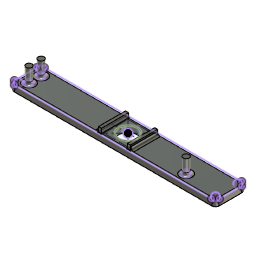
Front_Cover_OV3660 (Autodesk Fusion 360 design; units mm, degrees)
Autodesk Fusion 360 part; units mm, degrees
imported_body "Base Feature1" makes body 1
sketch "sketch 169" plane through (0, 0, 2) normal (0, 0, 1) x (-1, 0, 0)
  line L0 (-67.2527, -0.8) -> (-67.2527, -8.2)
  arc A0 (-67.2527, -8.2) -> (-66, -9.4527) centre (-66, -8.2) ccw
  line L1 (-66, -9.4527) -> (-0.8, -9.4527)
  arc A1 (-0.8, -9.4527) -> (0.4527, -8.2) centre (-0.8, -8.2) ccw
  line L2 (0.4527, -8.2) -> (0.4527, -0.8)
  arc A2 (0.4527, -0.8) -> (-0.8, 0.4527) centre (-0.8, -0.8) ccw
  line L3 (-0.8, 0.4527) -> (-66, 0.4527)
  arc A3 (-66, 0.4527) -> (-67.2527, -0.8) centre (-66, -0.8) ccw
  line L4 (-12, -7.75) -> (-15, -7.75)
  line L5 (-37.8, 0) -> (-37.8, -9)
  line L6 (-37.8, -9) -> (-39.8, -9)
  line L7 (-67.2527, -0.8) -> (-67.2527, -8.2)
  arc A4 (-67.2527, -8.2) -> (-66, -9.4527) centre (-66, -8.2) ccw
  line L8 (-66, -9.4527) -> (-0.8, -9.4527)
  arc A5 (-0.8, -9.4527) -> (0.4527, -8.2) centre (-0.8, -8.2) ccw
  line L9 (0.4527, -8.2) -> (0.4527, -0.8)
  arc A6 (0.4527, -0.8) -> (-0.8, 0.4527) centre (-0.8, -0.8) ccw
  line L10 (-0.8, 0.4527) -> (-66, 0.4527)
  arc A7 (-66, 0.4527) -> (-67.2527, -0.8) centre (-66, -0.8) ccw
  line L11 (-0.8, 0.4527) -> (-66, 0.4527)
  line L12 (-67.2527, -0.8) -> (-67.2527, -8.2)
  line L13 (-66, -9.4527) -> (-0.8, -9.4527)
  line L14 (0.4527, -8.2) -> (0.4527, -0.8)
  arc A8 (-0.8, -9.4527) -> (0.4527, -8.2) centre (-0.8, -8.2) ccw
  arc A9 (0.4527, -0.8) -> (-0.8, 0.4527) centre (-0.8, -0.8) ccw
  arc A10 (-66, 0.4527) -> (-67.2527, -0.8) centre (-66, -0.8) ccw
  arc A11 (-67.2527, -8.2) -> (-66, -9.4527) centre (-66, -8.2) ccw
  line L15 (0.1, -0.5) -> (-60.4, -0.5) construction
  line L16 (-60.4, -0.5) -> (-60.4, -8.5) construction
  line L17 (-60.4, -8.5) -> (0.1, -8.5) construction
  line L18 (0.1, -8.5) -> (0.1, -0.5) construction
  circle A12 centre (-33.4, -4.5) radius 3.1
  line L19 (0.1, -4.5) -> (-60.4, -4.5) construction
  line L20 (-0.8, -8.2) -> (-66, -0.8) construction
  line L21 (-66, -8.2) -> (-0.8, -0.8) construction
  constraint coincident A2.end L3.start
  constraint coincident L3.end A3.start
  constraint coincident L0.start A3.end
  constraint coincident L0.end A0.start
  constraint coincident A0.end L1.start
  constraint coincident L1.end A1.start
  constraint coincident A1.end L2.start
  constraint coincident L2.end A2.start
  constraint tangent L8 A8
  constraint tangent L14 A9
  constraint tangent L11 A9
  constraint tangent L11 A10
  constraint tangent L12 A11
  constraint horizontal L15
  constraint vertical L16
  constraint horizontal L17
  constraint vertical L18
  constraint coincident L15.start L18.end
  constraint midpoint L18 L19.start
  constraint midpoint L16 L19.end
  constraint coincident A12.centre L19
  constraint coincident A1.centre A5.centre
  constraint coincident A3.centre A7.centre
  constraint coincident A0.centre A4.centre
  constraint coincident A2.centre A6.centre
  constraint coincident A12.centre L21
  constraint coincident A12.centre L20
extrude "Extrude1" add sketch "sketch 169" against normal blind 2 separate body makes body 2
sketch "sketch 484" plane through (0, 0, 2) normal (0, 0, 1) x (-1, 0, 0)
  arc A0 (-67.2527, -8.2) -> (-66, -9.4527) centre (-66, -8.2) ccw
  line L0 (-66, -9.4527) -> (-0.8, -9.4527)
  arc A1 (-0.8, -9.4527) -> (0.4527, -8.2) centre (-0.8, -8.2) ccw
  line L1 (0.4527, -8.2) -> (0.4527, -0.8)
  arc A2 (0.4527, -0.8) -> (-0.8, 0.4527) centre (-0.8, -0.8) ccw
  line L2 (-0.8, 0.4527) -> (-66, 0.4527)
  arc A3 (-66, 0.4527) -> (-67.2527, -0.8) centre (-66, -0.8) ccw
  line L3 (-67.2527, -0.8) -> (-67.2527, -8.2)
  circle A4 centre (-33.5, -4.25) radius 3.1
  circle A5 centre (-2.7, -2.5) radius 1
  circle A6 centre (-2.7, -6.5) radius 1
  line L4 (-2.7, -2.5) -> (-2.7, -6.5) construction
  line L5 (-4.05, -4.5) -> (-64.55, -4.5) construction
  circle A7 centre (-54.6, -2.5) radius 1
  line L6 (-2.7, -2.5) -> (-54.6, -2.5) construction
  line L7 (-60.4, -0.5) -> (-60.4, -8.5) construction
  line L8 (0.1, -8.5) -> (0.1, -0.5) construction
  line L9 (0.1, -4.5) -> (-60.4, -4.5) construction
  constraint equal A5 A6
  constraint coincident A5.centre L4.start
  constraint coincident A6.centre L4.end
  constraint vertical L4
  constraint equal A6 A7
  constraint coincident A7.centre L6.end
  constraint horizontal L6
  constraint collinear L5 L9
extrude "Extrude2" add sketch "sketch 484" along normal blind 5 contours A5 | A6 | A7 bodies 2
sketch "Sketch1" plane through (0, 0, 2) normal (0, 0, 1) x (1, 0, 0)
  circle A0 centre (33.4, 4.5) radius 3.1
  line L0 (29.4, 8.5) -> (37.4, 8.5) construction
  line L1 (37.4, 8.5) -> (37.4, 0.5) construction
  line L2 (37.4, 0.5) -> (29.4, 0.5) construction
  line L3 (29.4, 0.5) -> (29.4, 8.5) construction
  line L4 (29.4, 8.5) -> (37.4, 0.5) construction
  line L5 (37.4, 8.5) -> (29.4, 0.5) construction
  line L6 (29.1, 0) -> (28.1, 0)
  line L7 (28.1, 0) -> (28.1, 9)
  line L8 (28.1, 9) -> (29.1, 9)
  line L9 (29.1, 9) -> (29.1, 0)
  line L10 (38.7, 0) -> (37.7, 0)
  line L11 (37.7, 0) -> (37.7, 9)
  line L12 (37.7, 9) -> (38.7, 9)
  line L13 (38.7, 9) -> (38.7, 0)
  line L14 (28.1, 4.5) -> (37.7, 4.5) construction
  circle A1 centre (54.6, 2.5) radius 1
  circle A2 centre (2.7, 2.5) radius 1
  circle A3 centre (2.7, 6.5) radius 1
  circle A4 centre (33.4, 4.5) radius 3.1
  arc A5 (67.2527, 8.2) -> (66, 9.4527) centre (66, 8.2) ccw
  line L15 (66, 9.4527) -> (0.8, 9.4527)
  arc A6 (0.8, 9.4527) -> (-0.4527, 8.2) centre (0.8, 8.2) ccw
  line L16 (-0.4527, 8.2) -> (-0.4527, 0.8)
  arc A7 (-0.4527, 0.8) -> (0.8, -0.4527) centre (0.8, 0.8) ccw
  line L17 (0.8, -0.4527) -> (66, -0.4527)
  arc A8 (66, -0.4527) -> (67.2527, 0.8) centre (66, 0.8) ccw
  line L18 (67.2527, 0.8) -> (67.2527, 8.2)
  point P0 (33.4, 4.5)
  dimension "d5" = 8
  dimension "d6" = 8
  dimension "d7" = 1
  dimension "d8" = 0.3
  dimension "d9" = 0.3
  dimension "d10" = 9
  constraint horizontal L0
  constraint perpendicular L0 L1
  constraint parallel L0 L2
  constraint parallel L1 L3
  constraint coincident L4 P0
  constraint coincident L5 P0
  constraint coincident P0 A0.centre
  constraint horizontal L6
  constraint vertical L7
  constraint horizontal L8
  constraint vertical L9
  constraint horizontal L10
  constraint vertical L11
  constraint horizontal L12
  constraint vertical L13
  constraint equal L6 L10
  constraint midpoint L7 L14.start
  constraint midpoint L11 L14.end
  constraint coincident P0 L14
  constraint horizontal L14
  constraint equal L7 L13
  measures "d5" distance of L1.end L2.end
  measures "d6" distance of L0.end L1.end
  measures "d7" distance of L10.start L10.end
  measures "d8" distance of L1 L11
  measures "d9" distance of L3 L9
  measures "d10" distance of L6.end L7.end
extrude "Extrude3" add sketch "Sketch1" along normal blind 1.5 contours L6 L7 L8 L9 | L10 L11 L12 L13 bodies 2
chamfer "Chamfer1" distance 0.5 distance2 2 8 edges at (33.4, 9.4527, 2) (-0.0858, 9.0858, 2) (-0.4527, 4.5, 2) (-0.0858, -0.0858, 2) (33.4, -0.4527, 2) (66.8858, -0.0858, 2) (67.2527, 4.5, 2) (66.8858, 9.0858, 2) measured on face at (19.9629, 3.883, 2) measured on face at (19.9629, 3.883, 2) measured on face at (19.9629, 3.883, 2) measured on face at (19.9629, 3.883, 2) measured on face at (19.9629, 3.883, 2) measured on face at (19.9629, 3.883, 2) measured on face at (19.9629, 3.883, 2) measured on face at (19.9629, 3.883, 2) on bodies 2
fillet "Fillet1" radius 1 5 edges at (38.7, 4.5, 2) (55.5323, 2.1384, 2) (3.6323, 6.1384, 2) (3.6323, 2.1384, 2) (28.1, 4.5, 2) on bodies 2
sketch "sketch 731" plane through (0, 0, 0) normal (0, 0, -1) x (1, 0, 0)
  line L0 (53.3865, -6.5641) -> (49.9223, -8.5639)
  line L1 (49.9223, -8.5639) -> (46.4583, -6.5637)
  line L2 (46.4583, -6.5637) -> (46.4586, -2.5637)
  line L3 (46.4586, -2.5637) -> (49.9228, -0.5639)
  line L4 (49.9228, -0.5639) -> (53.3868, -2.5641)
  line L5 (53.3868, -2.5641) -> (53.3865, -6.5641)
  line L6 (49.6975, -2.3559) -> (48.6975, -2.3558)
  line L7 (48.6975, -2.3558) -> (47.4226, -4.5637)
  line L8 (47.4226, -4.5637) -> (48.4226, -4.5638)
  line L9 (48.4226, -4.5638) -> (49.6975, -2.3559)
  line L10 (50.6975, -2.3559) -> (48.1477, -6.7718)
  line L11 (51.6975, -2.356) -> (50.6975, -2.3559)
  line L12 (49.1476, -6.7718) -> (51.6975, -2.356)
  line L13 (48.1477, -6.7718) -> (49.1476, -6.7718)
  line L14 (51.4225, -4.564) -> (50.1476, -6.7719)
  line L15 (52.4225, -4.564) -> (51.4225, -4.564)
  line L16 (51.1476, -6.772) -> (52.4225, -4.564)
  line L17 (50.1476, -6.7719) -> (51.1476, -6.772)
extrude "Extrude4" cut sketch "sketch 731" against normal blind 0.4 bodies 2
hidden bodies 1
